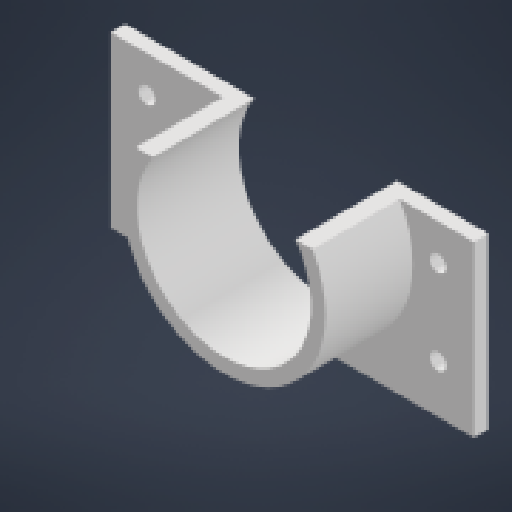
# Autodesk Inventor part: Rex Motor Bracket
Saved by Autodesk Inventor 2023 (Build 270158000, 158)
## iProperties
Created: 2022-12-08
Part Number: Rex Motor Bracket
Material: Generic
Document SubType Name: Modeling
Designer: Izack Waczko
Density: 1 g/cm^3
Appearance: Default
Author: Izack Waczko
Autodesk Inventor part; units mm, degrees
ref_plane "YZ Plane" through (0, 0, 0) normal (1, 0, 0) x (0, 1, 0)
ref_plane "XZ Plane" through (0, 0, 0) normal (0, 1, 0) x (-1, 0, 0)
ref_plane "XY Plane" through (0, 0, 0) normal (0, 0, 1) x (1, 0, 0)
sketch "Sketch1" plane through (0, 0, 0) normal (0, 0, 1) x (1, 0, 0)
  circle A0 centre (-15, 75) radius 1.7 projected
  circle A1 centre (-15, 57.5) radius 1.7 projected
  circle A2 centre (-75, 75) radius 1.7 projected
  circle A3 centre (-75, 57.5) radius 1.7 projected
  line L0 (-67.5, 62.5) -> (-67.5, 82.5) projected
  arc A4 (-67.5, 62.5) -> (-57.5, 52.5) centre (-57.5, 62.5) ccw projected
  line L1 (-32.5, 52.5) -> (-57.5, 52.5) projected
  arc A5 (-32.5, 52.5) -> (-22.5, 62.5) centre (-32.5, 62.5) ccw projected
  line L2 (-22.5, 82.5) -> (-22.5, 62.5) projected
  line L3 (-7.5, 82.5) -> (-22.5, 82.5) projected
  line L4 (-7.5, 62.5) -> (-7.5, 82.5) projected
  line L5 (-67.5, 82.5) -> (-82.5, 82.5) projected
  line L6 (-82.5, 82.5) -> (-82.5, -37.5) projected
  line L7 (-82.5, 52.5) -> (-57.5, 52.5)
  line L8 (-32.5, 52.5) -> (-7.5, 52.5)
  line L9 (-7.5, 52.5) -> (-7.5, 62.5)
  circle A6 centre (-41.0876, 72.1294) radius 17.98 projected
  line L10 (-67.5, 82.5) -> (-55.7753, 82.5)
  line L11 (-22.5, 82.5) -> (-26.3998, 82.5)
  line L12 (-7.5, 52.5) -> (-82.5, 52.5)
  line L13 (-82.5, 52.5) -> (-82.5, 47.5)
  line L14 (-82.5, 47.5) -> (-7.5, 47.5)
  line L15 (-7.5, 47.5) -> (-7.5, 52.5)
  point P0 (0, 0)
  point P1 (-22.2961, 67.9529)
  dimension "d2" = 5
  constraints: 18 end point, 4 point on line, 3 perpendicular, 3 point on circle, 2 horizontal, 2 parallel, 1 other
  measures "d2" distance of L13.end L12.end
extrude "Extrusion1" add sketch "Sketch1" along normal blind 3 contours A4 L7 L6 L5 L0 | L0 L10 A6 L11 L2 A5 L1 A4 | L1 L8 L15 L14 L6 L7 | A5 L2 L3 L4 L9 L8
sketch "Sketch2" plane through (0, 0, 3) normal (0, 0, 1) x (1, 0, 0)
  circle A0 centre (-41.0876, 72.1294) radius 17.98 projected
  line L0 (-55.7753, 82.5) -> (-82.5, 82.5) projected
  line L1 (-7.5, 82.5) -> (-26.3998, 82.5) projected
  circle A1 centre (-41.0876, 72.1294) radius 23.98
  point P0 (0, 0)
  point P1 (-62.7091, 82.5)
  point P2 (-19.466, 82.5)
  dimension "d3" = 6
  constraints: 1 centre point
  measures "d3" radial gap between concentric circles of A0 A1
ref_plane "Work Plane1" through (-53.7982, 52.0166, 21) normal (0, 0, 1) x (0.817541, 0.5758704, 0)
extrude "Extrusion2" add sketch "Sketch2" along normal up to surface (18 mm away) contours A0 L1 A1 L0 picked at (-19.4997, 68.841)
sketch "Sketch3" plane through (-41.0876, 72.1294, 21) normal (0, 0, 1) x (1, 0, 0)
  arc A0 (-21.6215, 10.3706) -> (21.6215, 10.3706) centre (0, 0) ccw projected
  circle A1 centre (0, 0) radius 4.485 projected
  arc A2 (-14.6878, 10.3706) -> (14.6878, 10.3706) centre (0, 0) ccw construction
  circle A3 centre (0, 0) radius 11.3137 construction
  point P0 (41.0876, -72.1294)
  constraints: 1 centre point, 1 coincident
body "Solid1"
